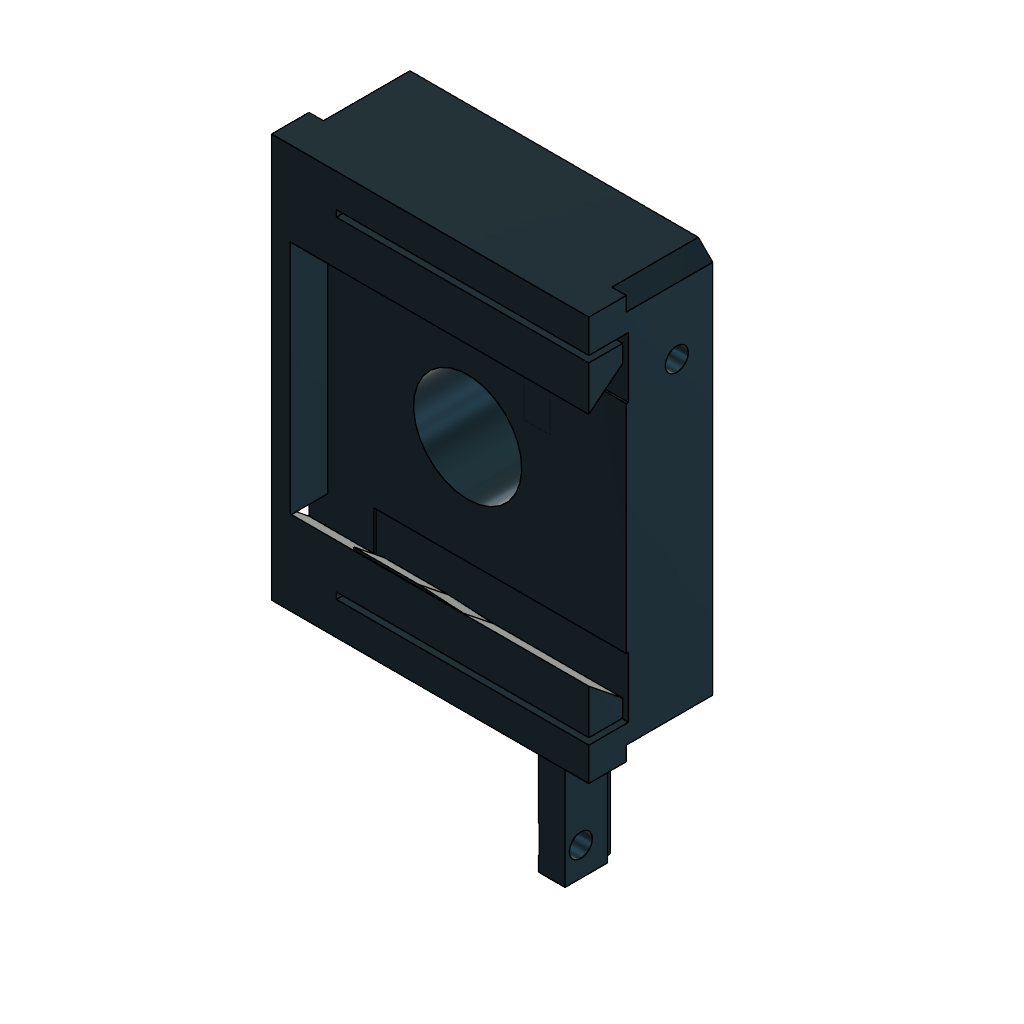
receiver_heat_stake (Autodesk Fusion 360 design; units mm, degrees)
part number: 2026-10-03-14-01-57-908
Autodesk Fusion 360 part; units mm, degrees
ref_plane "工作平面1" through (0, 0, 0) normal (0, 0, 1) x (1, 0, 0)
sketch "草图1" plane through (0, 0, 0) normal (0, 0, 1) x (1, 0, 0)
  line L0 (-26, -22) -> (26, -22)
  line L1 (26, -22) -> (28, -20)
  line L2 (28, -20) -> (28, 20)
  line L3 (28, 20) -> (26, 22)
  line L4 (26, 22) -> (-26, 22)
  line L5 (-26, 22) -> (-28, 20)
  line L6 (-28, 20) -> (-28, -20)
  line L7 (-28, -20) -> (-26, -22)
extrude "56 x 44 x 7 platform" add sketch "草图1" along normal blind 12
ref_plane "工作平面2" through (0, 0, 12) normal (0, 0, 1) x (1, 0, 0)
sketch "草图2" plane through (0, 0, 12) normal (0, 0, 1) x (1, 0, 0)
  line L0 (-28, -22) -> (-20.49, -22)
  line L1 (-20.49, -22) -> (-20.49, 22)
  line L2 (-20.49, 22) -> (-28, 22)
  line L3 (-28, 22) -> (-28, -22)
ref_plane "工作平面3" through (0, 0, 17.2) normal (0, 0, 1) x (1, 0, 0)
sketch "草图3" plane through (0, 0, 17.2) normal (0, 0, 1) x (1, 0, 0)
  line L0 (-28, -22) -> (-16.33, -22)
  line L1 (-16.33, -22) -> (-16.33, 22)
  line L2 (-16.33, 22) -> (-28, 22)
  line L3 (-28, 22) -> (-28, -22)
loft "Dovetail retaining rail 0.8 to 1 -1" add profiles "草图2", "草图3" section 1 section 2
ref_plane "工作平面4" through (0, 0, 11.7) normal (0, 0, 1) x (1, 0, 0)
sketch "草图4" plane through (0, 0, 11.7) normal (0, 0, 1) x (1, 0, 0)
  line L0 (-23.4, -22) -> (-22.5, -22)
  line L1 (-22.5, -22) -> (-22.5, 13)
  line L2 (-22.5, 13) -> (-23.4, 13)
  line L3 (-23.4, 13) -> (-23.4, -22)
extrude "0.9 mm longitudinal flexure slot -1" cut sketch "草图4" along normal blind 5.8
ref_plane "工作平面5" through (0, 0, 11.7) normal (0, 0, 1) x (1, 0, 0)
sketch "草图5" plane through (0, 0, 11.7) normal (0, 0, 1) x (1, 0, 0)
  line L0 (-22.5, -22) -> (-15, -22)
  line L1 (-15, -22) -> (-15, 13)
  line L2 (-15, 13) -> (-22.5, 13)
  line L3 (-22.5, 13) -> (-22.5, -22)
extrude "0.8 mm flexure underside relief -1" cut sketch "草图5" along normal blind 0.8
ref_plane "工作平面6" through (0, 0, 12.6) normal (0, 0, 1) x (1, 0, 0)
sketch "草图6" plane through (0, 0, 12.6) normal (0, 0, 1) x (1, 0, 0)
  line L0 (-20.21, -6) -> (-20.21, 11)
  line L1 (-20.21, 11) -> (-19.66, 11)
  line L2 (-19.66, 11) -> (-19.66, 2)
  line L3 (-19.66, 2) -> (-20.11, -6)
  line L4 (-20.11, -6) -> (-20.21, -6)
ref_plane "工作平面7" through (0, 0, 16.8) normal (0, 0, 1) x (1, 0, 0)
sketch "草图7" plane through (0, 0, 16.8) normal (0, 0, 1) x (1, 0, 0)
  line L0 (-16.85, -6) -> (-16.85, 11)
  line L1 (-16.85, 11) -> (-16.3, 11)
  line L2 (-16.3, 11) -> (-16.3, 2)
  line L3 (-16.3, 2) -> (-16.75, -6)
  line L4 (-16.75, -6) -> (-16.85, -6)
loft "Tapered friction contact rib -1" add profiles "草图6", "草图7" section 1 section 2
ref_plane "工作平面8" through (0, 0, 12) normal (0, 0, 1) x (1, 0, 0)
sketch "草图8" plane through (0, 0, 12) normal (0, 0, 1) x (1, 0, 0)
  line L0 (20.49, -22) -> (28, -22)
  line L1 (28, -22) -> (28, 22)
  line L2 (28, 22) -> (20.49, 22)
  line L3 (20.49, 22) -> (20.49, -22)
ref_plane "工作平面9" through (0, 0, 17.2) normal (0, 0, 1) x (1, 0, 0)
sketch "草图9" plane through (0, 0, 17.2) normal (0, 0, 1) x (1, 0, 0)
  line L0 (16.33, -22) -> (28, -22)
  line L1 (28, -22) -> (28, 22)
  line L2 (28, 22) -> (16.33, 22)
  line L3 (16.33, 22) -> (16.33, -22)
loft "Dovetail retaining rail 0.8 to 1 1" add profiles "草图8", "草图9" section 1 section 2
ref_plane "工作平面10" through (0, 0, 11.7) normal (0, 0, 1) x (1, 0, 0)
sketch "草图10" plane through (0, 0, 11.7) normal (0, 0, 1) x (1, 0, 0)
  line L0 (22.5, -22) -> (23.4, -22)
  line L1 (23.4, -22) -> (23.4, 13)
  line L2 (23.4, 13) -> (22.5, 13)
  line L3 (22.5, 13) -> (22.5, -22)
extrude "0.9 mm longitudinal flexure slot 1" cut sketch "草图10" along normal blind 5.8
ref_plane "工作平面11" through (0, 0, 11.7) normal (0, 0, 1) x (1, 0, 0)
sketch "草图11" plane through (0, 0, 11.7) normal (0, 0, 1) x (1, 0, 0)
  line L0 (15, -22) -> (22.5, -22)
  line L1 (22.5, -22) -> (22.5, 13)
  line L2 (22.5, 13) -> (15, 13)
  line L3 (15, 13) -> (15, -22)
extrude "0.8 mm flexure underside relief 1" cut sketch "草图11" along normal blind 0.8
ref_plane "工作平面12" through (0, 0, 12.6) normal (0, 0, 1) x (1, 0, 0)
sketch "草图12" plane through (0, 0, 12.6) normal (0, 0, 1) x (1, 0, 0)
  line L0 (20.21, -6) -> (20.21, 11)
  line L1 (20.21, 11) -> (19.66, 11)
  line L2 (19.66, 11) -> (19.66, 2)
  line L3 (19.66, 2) -> (20.11, -6)
  line L4 (20.11, -6) -> (20.21, -6)
ref_plane "工作平面13" through (0, 0, 16.8) normal (0, 0, 1) x (1, 0, 0)
sketch "草图13" plane through (0, 0, 16.8) normal (0, 0, 1) x (1, 0, 0)
  line L0 (16.85, -6) -> (16.85, 11)
  line L1 (16.85, 11) -> (16.3, 11)
  line L2 (16.3, 11) -> (16.3, 2)
  line L3 (16.3, 2) -> (16.75, -6)
  line L4 (16.75, -6) -> (16.85, -6)
loft "Tapered friction contact rib 1" add profiles "草图12", "草图13" section 1 section 2
ref_plane "工作平面14" through (0, 0, 12) normal (0, 0, 1) x (1, 0, 0)
sketch "草图14" plane through (0, 0, 12) normal (0, 0, 1) x (1, 0, 0)
  line L0 (-16.5, 19.4) -> (16.5, 19.4)
  line L1 (16.5, 19.4) -> (16.5, 22)
  line L2 (16.5, 22) -> (-16.5, 22)
  line L3 (-16.5, 22) -> (-16.5, 19.4)
extrude "Closed insertion end stop" add sketch "草图14" along normal blind 5.2
ref_plane "工作平面15" through (0, 0, 0) normal (0, 0, 1) x (1, 0, 0)
sketch "草图15" plane through (0, 0, 0) normal (0, 0, 1) x (1, 0, 0)
  circle A0 centre (0, 0) radius 7.5
extrude "15 mm screw and driver access" cut sketch "草图15" along normal blind 12
move_body "Align camera long edge with gimbal arm - 90 degrees" bodies 1 to x (0, 1, 0) y (-1, 0, 0) z (0, 0, 1) at (0, 0, 0)
ref_plane "工作平面16" through (0, 0, 0) normal (0, 0, 1) x (1, 0, 0)
sketch "草图16" plane through (0, 0, 0) normal (0, 0, 1) x (1, 0, 0)
  line L0 (7.8, 5.95) -> (11.4, 5.95)
  line L1 (11.4, 5.95) -> (11.4, 21.05)
  line L2 (11.4, 21.05) -> (7.8, 21.05)
  line L3 (7.8, 21.05) -> (7.8, 5.95)
extrude "Clear original raised tab and root fillet" cut sketch "草图16" along normal blind 11.9
ref_plane "工作平面17" through (0, 0, -2.1) normal (0, 0, 1) x (1, 0, 0)
sketch "草图17" plane through (0, 0, -2.1) normal (0, 0, 1) x (1, 0, 0)
  line L0 (-8.5, -20) -> (-6.3, -20)
  line L1 (-6.3, -20) -> (-6.3, 20)
  line L2 (-6.3, 20) -> (-8.5, 20)
  line L3 (-8.5, 20) -> (-8.5, -20)
extrude "Arm lateral locating shoulder" add sketch "草图17" along normal blind 2.1
ref_plane "工作平面18" through (0, 0, -2.1) normal (0, 0, 1) x (1, 0, 0)
sketch "草图18" plane through (0, 0, -2.1) normal (0, 0, 1) x (1, 0, 0)
  line L0 (8.3, -20) -> (10.5, -20)
  line L1 (10.5, -20) -> (10.5, 20)
  line L2 (10.5, 20) -> (8.3, 20)
  line L3 (8.3, 20) -> (8.3, -20)
extrude "Arm lateral locating shoulder (1)" add sketch "草图18" along normal blind 2.1
ref_plane "工作平面19" through (0, 0, -5.5) normal (0, 0, 1) x (1, 0, 0)
sketch "草图19" plane through (0, 0, -5.5) normal (0, 0, 1) x (1, 0, 0)
  circle A0 centre (0, -24) radius 1.1
extrude "Reinforced 2.2 x 5.5 mm heat stake pin at arm y -4" add sketch "草图19" along normal blind 5.5
ref_plane "工作平面20" through (0, 0, -5.5) normal (0, 0, 1) x (1, 0, 0)
sketch "草图20" plane through (0, 0, -5.5) normal (0, 0, 1) x (1, 0, 0)
  circle A0 centre (0, -16) radius 1.1
extrude "Reinforced 2.2 x 5.5 mm heat stake pin at arm y 4" add sketch "草图20" along normal blind 5.5
ref_plane "工作平面21" through (0, 0, -5.5) normal (0, 0, 1) x (1, 0, 0)
sketch "草图21" plane through (0, 0, -5.5) normal (0, 0, 1) x (1, 0, 0)
  circle A0 centre (0, -10) radius 1.1
extrude "Reinforced 2.2 x 5.5 mm heat stake pin at arm y 10" add sketch "草图21" along normal blind 5.5
ref_plane "工作平面22" through (0, 0, -5.5) normal (0, 0, 1) x (1, 0, 0)
sketch "草图22" plane through (0, 0, -5.5) normal (0, 0, 1) x (1, 0, 0)
  circle A0 centre (0, 12) radius 1.1
extrude "Reinforced 2.2 x 5.5 mm heat stake pin at arm y 32" add sketch "草图22" along normal blind 5.5
ref_plane "工作平面23" through (0, 0, 0) normal (0, 0, 1) x (1, 0, 0)
sketch "草图23" plane through (0, 0, 0) normal (0, 0, 1) x (1, 0, 0)
  line L0 (5, -52.15) -> (8.7, -52.15)
  line L1 (8.7, -52.15) -> (8.7, -27.5)
  line L2 (8.7, -27.5) -> (5, -27.5)
  line L3 (5, -27.5) -> (5, -52.15)
extrude "Ear for original 3.2 mm side hole at arm y -28.15" add sketch "草图23" along normal blind 7.2
ref_plane "工作平面24" through (0, 0, 0) normal (0, 0, 1) x (1, 0, 0)
sketch "草图24" plane through (0, 0, 0) normal (0, 0, 1) x (1, 0, 0)
  line L0 (7.8, -52.15) -> (8.9, -52.15)
  line L1 (8.9, -52.15) -> (8.9, -27.5)
  line L2 (8.9, -27.5) -> (7.8, -27.5)
  line L3 (7.8, -27.5) -> (7.8, -52.15)
extrude "Ear relief around original arm root radius" cut sketch "草图24" along normal blind 1.3
ref_plane "工作平面25" through (4.9, 0, 0) normal (1, 0, 0) x (0, 1, 0)
sketch "草图25" plane through (4.9, 0, 0) normal (1, 0, 0) x (0, 0, -1)
  circle A0 centre (-5, -48.15) radius 1.6
extrude "Side rivet full passage clearance" cut sketch "草图25" along normal blind 20
ref_plane "工作平面26" through (2.9, 0, 0) normal (1, 0, 0) x (0, 1, 0)
sketch "草图26" plane through (2.9, 0, 0) normal (1, 0, 0) x (0, 0, -1)
  circle A0 centre (-5, -48.15) radius 2.9
extrude "Side rivet flange counterbore" cut sketch "草图26" along normal blind 2.2
ref_plane "工作平面27" through (0, 0, 0) normal (0, 0, 1) x (1, 0, 0)
sketch "草图27" plane through (0, 0, 0) normal (0, 0, 1) x (1, 0, 0)
  line L0 (5, 12.85) -> (8.7, 12.85)
  line L1 (8.7, 12.85) -> (8.7, 20.85)
  line L2 (8.7, 20.85) -> (5, 20.85)
  line L3 (5, 20.85) -> (5, 12.85)
extrude "Ear for original 3.2 mm side hole at arm y 36.85" add sketch "草图27" along normal blind 7.2
ref_plane "工作平面28" through (0, 0, 0) normal (0, 0, 1) x (1, 0, 0)
sketch "草图28" plane through (0, 0, 0) normal (0, 0, 1) x (1, 0, 0)
  line L0 (7.8, 12.85) -> (8.9, 12.85)
  line L1 (8.9, 12.85) -> (8.9, 20.85)
  line L2 (8.9, 20.85) -> (7.8, 20.85)
  line L3 (7.8, 20.85) -> (7.8, 12.85)
extrude "Ear relief around original arm root radius (1)" cut sketch "草图28" along normal blind 1.3
ref_plane "工作平面29" through (4.9, 0, 0) normal (1, 0, 0) x (0, 1, 0)
sketch "草图29" plane through (4.9, 0, 0) normal (1, 0, 0) x (0, 0, -1)
  circle A0 centre (-5, 16.85) radius 1.6
extrude "Side rivet full passage clearance (1)" cut sketch "草图29" along normal blind 20
ref_plane "工作平面30" through (2.9, 0, 0) normal (1, 0, 0) x (0, 1, 0)
sketch "草图30" plane through (2.9, 0, 0) normal (1, 0, 0) x (0, 0, -1)
  circle A0 centre (-5, 16.85) radius 2.9
extrude "Side rivet flange counterbore (1)" cut sketch "草图30" along normal blind 2.2
move_body "Move outward toward free end 20.0 mm" bodies 1 to x (1, 0, 0) y (0, 1, 0) z (0, 0, 1) at (0, 20, 0)
ref_plane "工作平面31" through (0, 0, -2.11) normal (0, 0, 1) x (1, 0, 0)
sketch "草图31" plane through (0, 0, -2.11) normal (0, 0, 1) x (1, 0, 0)
  line L0 (8.29, 25.95) -> (10.51, 25.95)
  line L1 (10.51, 25.95) -> (10.51, 40.05)
  line L2 (10.51, 40.05) -> (8.29, 40.05)
  line L3 (8.29, 40.05) -> (8.29, 25.95)
extrude "Trim locating shoulder before raised side ear root" cut sketch "草图31" along normal blind 2.11
named bodies: "Receiver_heat_stake_optimized"
